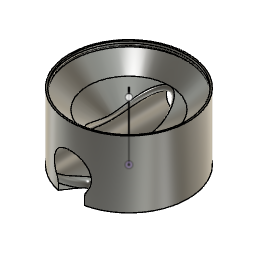
Base (Autodesk Fusion 360 design; units mm, degrees)
Autodesk Fusion 360 part; units mm, degrees
note: some values were not read from the file. Set by a fixed rule: which sketch regions a step uses.
sketch "Sketch1" plane through (0, 0, 0) normal (0, 0, 1) x (1, 0, 0)
  circle A0 centre (0, 0) radius 57.5
  line L0 (0, 0) -> (47.5, 0) construction
  line L1 (0, 0) -> (47.5, 0) construction
  line L2 (0, 0) -> (47.5, 0) construction
  line L3 (0, 0) -> (47.5, 0) construction
  circle A1 centre (-33.5876, -33.5876) radius 2.15
  circle A2 centre (33.5876, -33.5876) radius 2.15
  circle A3 centre (33.5876, 33.5876) radius 2.15
  circle A4 centre (-33.5876, 33.5876) radius 2.15
  spline S0 degree 2 poles (-12.8388, -56.0483) (0, -36) (12.5423, -56.1154) knots 0 0 0 4.029531 4.029531 4.029531 weights 1 3.529401 1
  dimension "d1" = 115
  dimension "d26" = 4.3
  dimension "d27" = 4.3
  dimension "d28" = 4.3
  dimension "d29" = 4.3
  constraint coincident A0.centre L0.start
  constraint horizontal L0
  constraint horizontal L1
  constraint horizontal L2
  constraint horizontal L3
  constraint coincident A0 S0.end
  constraint coincident A0 S0.start
  measures "d1" diameter of A0
  measures "d26" diameter of A1
  measures "d27" diameter of A2
  measures "d28" diameter of A3
  measures "d29" diameter of A4
extrude "Extrude1" add sketch "Sketch1" along normal blind 60 contours A0 S0 | A0 S0 | A1 | A2 | A3 | A4
sketch "Sketch2" plane through (0, 0, 0) normal (0, 1, 0) x (1, 0, 0)
  line L0 (0, 0) -> (0, -5)
  line L1 (0, -5) -> (0, -41)
  circle A0 centre (0, -23) radius 18
  circle A1 centre (0, -23) radius 25
  dimension "d4" = 5
  dimension "d5" = 36
  dimension "d17" = 50
  constraint coincident L0.start origin
  constraint vertical L0
  constraint parallel L0 L1
  constraint coincident L1.end A0
  constraint coincident L0.end A0
  constraint concentric A0 A1
  measures "d4" distance of L0.start L0.end
  measures "d5" distance of L0.end L1.end
  measures "d17" diameter of A1
extrude "Extrude2" cut sketch "Sketch2" along normal mid plane 120 contours L1 A0 | L1 A0
hole "Hole1" at (0, 0, 60) direction (0, 0, -1) diameter 80 depth 13.4256 tip angle 118 countersink diameter 112 countersink angle 100
fillet "Fillet1" radius 3 1 edges at (-15.6284, 0, 31.9305)
extrude "Extrude3" add 1 faces at (-46.5962, -31.7688, 60) along direction (0, 0, 1) blind 5
sketch "Sketch3" plane through (0, 0, 0) normal (0, 0, 1) x (1, 0, 0)
sketch "Sketch4" plane through (0, 0, 0) normal (0, 0, 1) x (1, 0, 0)
extrude "Extrude4" cut sketch "Sketch1" along normal blind 5.5 contours A1 | A2 | A3 | A4
extrude "Extrude5" cut sketch "Sketch1" along normal blind 12 contours A0 S0 picked at (-0.6262, -48.921)
fillet "Fillet2" radius 7 1 edges at (-0.2876, -40.4473, 5.0023)
sketch "Sketch5" plane through (0, 0, 0) normal (0, 1, 0) x (1, 0, 0)
  line L0 (0, 0) -> (0, -65)
  line L1 (0, -65) -> (0, -57)
  dimension "d38" = 8
  constraint coincident L0.start origin
  constraint vertical L0
  constraint parallel L0 L1
  measures "d38" distance of L0.end L1.end
ref_plane "WorkPlane1" through (0, 0, 61) normal (0, 0, 1) x (1, 0, 0)
coil "CoilPrimitive1" add diameter 112 section circle size 1.5 on centre turns 1 pitch 3 right hand placed x (1, 0, 0) y (0, 1, 0) z (0, 0, 1) at (0, 0, 61)
fillet "Fillet3" radius 0.73 2 edges at (55.25, 0, 61) (55.25, 0, 64)
